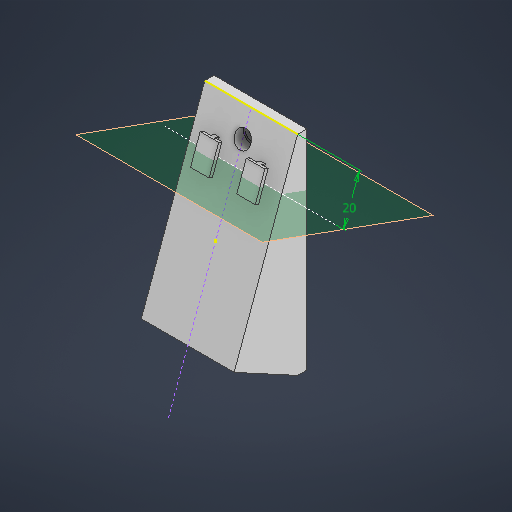
# Autodesk Inventor part: LCD_Mount_20degrees
Saved by Autodesk Inventor 2026.2 (Build 302298010, 298A)
## iProperties
Created: 2026-08-14
Part Number: LCD_Mount_20degrees
Material: 일반
Document SubType Name: Modeling
Designer: User
Density: 1 g/cm^3
Appearance: 기본값
Author: User
Autodesk Inventor part; units mm, degrees
ref_plane "YZ Plane" through (0, 0, 0) normal (1, 0, 0) x (0, 1, 0)
ref_plane "XZ Plane" through (0, 0, 0) normal (0, 1, 0) x (-1, 0, 0)
sketch "스케치2" plane through (0, 0, 0) normal (1, 0, 0) x (0, 1, 0)
  line L0 (-42.3529, 0) -> (47.6471, 0) construction
  line L1 (47.6471, 0) -> (-27.5284, 27.3616)
  line L2 (-27.5284, 27.3616) -> (-42.3529, 0)
  line L3 (47.6471, 0) -> (-42.3529, 0) construction
  line L4 (-42.3529, 0) -> (-42.3529, -4)
  line L5 (-42.3529, -4) -> (47.6471, -4)
  line L6 (47.6471, -4) -> (47.6471, 0)
  point P0 (0, 0)
  dimension "d2" = 90
  dimension "d3" = 80
  dimension "d4" = 20
  dimension "d7" = 4
  constraints: 14 end point, 2 horizontal, 2 parallel, 1 perpendicular
  measures "d2" distance of L0.start L0.end
  measures "d3" distance of L0.end L1.end
  measures "d4" angle of L0 L1
  measures "d7" distance of L3.end L4.end
extrude "돌출2" add sketch "스케치2" along normal mid plane 40
sketch "스케치3" plane through (20, 47.6471, -4) normal (0, 0, -1) x (-1, 0, 0)
  line L0 (40, 0) -> (0, 0) projected
  line L1 (0, -10) -> (40, -10)
  line L2 (40, -90) -> (0, -90) projected
  line L3 (0, -75.1754) -> (0, -90) projected
  line L4 (0, -80) -> (40, -80)
  line L5 (40, 0) -> (40, -90) projected
  line L6 (20, -93) -> (20, 7) construction
  circle A0 centre (20, -80) radius 2.5
  circle A1 centre (20, -10) radius 2.5
  point P0 (20, -47.6471)
  dimension "d10" = 10
  dimension "d12" = 10
  dimension "d13" = 5
  dimension "d14" = 5
  constraints: 6 end point, 4 point on line, 2 centre point, 2 horizontal, 2 midpoint, 1 vertical
  measures "d10" distance between parallel lines of L1 L0
  measures "d12" distance between parallel lines of L2 L4
  measures "d13" diameter of A0
  measures "d14" diameter of A1
extrude "돌출3" cut sketch "스케치3" against normal blind 40 contours A1 L1 | L1 A1 | A0 L4 | L4 A0
ref_plane "작업 평면3" through (0, 0, 27) normal (0, 0, 1) x (1, 0, 0)
sketch "스케치4" plane through (0, 0, 27) normal (0, 0, 1) x (1, 0, 0)
  circle A0 centre (0, 37.6471) radius 2.5 projected
  circle A1 centre (0, -32.3529) radius 2.5 projected
  circle A2 centre (0, 37.6471) radius 3.5
  circle A3 centre (0, -32.3529) radius 3.5
  point P0 (0, 0)
  dimension "d18" = 7
  dimension "d19" = 7
  constraints: 2 centre point, 2 coincident
  measures "d18" diameter of A2
  measures "d19" diameter of A3
extrude "돌출4" cut sketch "스케치4" against normal blind 27 contours A0 | A1 | A2 | A3
sketch "스케치5" plane through (-20, -27.5284, 27.3616) normal (0, 0.3420201, 0.9396926) x (1, 0, 0)
  line L0 (20, 80) -> (20, -25) construction
  line L1 (-10, 60) -> (63, 60) construction
  line L2 (0, 80) -> (40, 80) projected
  point P0 (20, 35.2264)
  dimension "d22" = 20
  constraints: 4 end point, 1 horizontal, 1 vertical
  measures "d22" distance between parallel lines of L1 L2
ref_plane "작업 평면4" through (-30, 28.8532, 6.8404) normal (0, -0.9396926, 0.3420201) x (1, 0, 0)
sketch "스케치6" plane through (-30, 28.8532, 6.8404) normal (0, -0.9396926, 0.3420201) x (1, 0, 0)
  line L0 (30, 15) -> (30, -51) construction
  line L1 (26.5, 0) -> (33.5, 0) projected
  line L2 (10, 0) -> (50, 0) projected
  line L3 (21, 0) -> (21, 0)
  line L4 (50, 0) -> (50, -30.7818) projected
  line L5 (19.1, 0) -> (21, 0)
  line L6 (21, 0) -> (21, 2)
  line L7 (19.1, 2) -> (19.1, 0)
  line L8 (16.05, 3.5) -> (24.05, 3.5)
  line L9 (24.05, 3.5) -> (24.05, 2)
  line L10 (16.05, 2) -> (16.05, 3.5)
  line L11 (24.05, 2) -> (21, 2)
  line L12 (19.1, 2) -> (16.05, 2)
  line L13 (39, 0) -> (39, 2)
  line L14 (40.9, 2) -> (40.9, 0)
  line L15 (43.95, 3.5) -> (35.95, 3.5)
  line L16 (35.95, 3.5) -> (35.95, 2)
  line L17 (43.95, 2) -> (43.95, 3.5)
  line L18 (35.95, 2) -> (39, 2)
  line L19 (40.9, 2) -> (43.95, 2)
  point P0 (30, -16.2963)
  point P1 (21, 1)
  point P2 (39, 1)
  point P3 (39, 0)
  point P4 (40.9, 0)
  dimension "d27" = 20
  dimension "d30" = 9
  dimension "d35" = 8
  dimension "d36" = 1.5
  dimension "d37" = 2
  dimension "d38" = 3.05
  constraints: 34 end point, 9 symmetric about line, 4 parallel, 3 horizontal, 2 perpendicular, 2 point on line, 1 midpoint, 1 vertical
  measures "d27" distance between parallel lines of L4 L0
  measures "d30" distance from line of L0 point (21, 1)
  measures "d35" distance of L8.start L8.end
  measures "d36" distance of L10.start L8.start
  measures "d37" distance of L7.start L5.start
  measures "d38" distance of L7.start L10.start
extrude "돌출5" add sketch "스케치6" along normal mid plane 12
